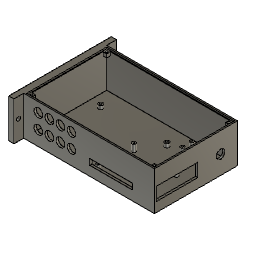
module_main v2 (Autodesk Fusion 360 design; units mm, degrees)
Autodesk Fusion 360 part; units mm, degrees
sketch "Sketch1" plane through (0, 0, 0) normal (0, 0, 1) x (1, 0, 0)
  line L0 (0, 0) -> (178, 0)
  line L1 (178, 0) -> (178, 113)
  line L2 (178, 113) -> (0, 113)
  line L3 (0, 113) -> (0, 0)
  dimension "d1" = 178
  dimension "d2" = 113
  constraint horizontal L0
  constraint vertical L1
  constraint horizontal L2
  constraint vertical L3
  constraint coincident L0.start L3.end
  measures "d1" distance of L0.start L0.end
  measures "d2" distance of L0.start L2.end
extrude "Extrude1" add sketch "Sketch1" along normal blind 3
extrude "Extrude2" add 1 faces at (59.3333, 37.6667, 3) along direction (0, 0, 1) blind 50 thin wall 3 inside
sketch "Sketch2" plane through (0, 0, 0) normal (-1, 0, 0) x (0, -1, 0)
  line L0 (-113, 0) -> (0, 0)
  line L1 (0, 0) -> (0, 53)
  line L2 (0, 53) -> (-113, 53)
  line L3 (-113, 53) -> (-113, 0)
  line L4 (13.35, 0) -> (-126.35, 0)
  line L5 (-126.35, 0) -> (-126.35, 53)
  line L6 (-126.35, 53) -> (13.35, 53)
  line L7 (13.35, 53) -> (13.35, 0)
  line L8 (13.35, 0) -> (-126.35, 53) construction
  line L9 (-126.35, 0) -> (13.35, 53) construction
  point P0 (-56.5, 26.5)
  dimension "d8" = 139.7
  dimension "d9" = 53
  constraint horizontal L4
  constraint perpendicular L4 L5
  constraint parallel L4 L6
  constraint parallel L5 L7
  constraint coincident L8 P0
  constraint coincident L9 P0
  measures "d8" distance of L5.end L6.end
  measures "d9" distance of L4.end L5.end
extrude "Extrude3" add sketch "Sketch2" along normal blind 7
sketch "Sketch3" plane through (-7, 0, 0) normal (-1, 0, 0) x (0, -1, 0)
  line L0 (13.35, 53) -> (-126.35, 53)
  line L1 (-126.35, 53) -> (-126.35, 0)
  line L2 (-126.35, 0) -> (13.35, 0)
  line L3 (13.35, 0) -> (13.35, 53)
  point P0 (-120, 26.5)
  point P1 (7, 26.5)
hole "Hole1" at (-7, 120, 26.5) at (-7, -7, 26.5) direction (1, 0, 0) diameter 5.5 depth 12 tip angle 118
sketch "Sketch4" plane through (0, 0, 3) normal (0, 0, 1) x (-1, 0, 0)
  line L0 (-175, -110) -> (-3, -110)
  line L1 (-3, -110) -> (-3, -3)
  line L2 (-3, -3) -> (-175, -3)
  line L3 (-175, -3) -> (-175, -110)
  circle A0 centre (-151.5, -7.5) radius 2.5
  circle A1 centre (-151.5, -56.5) radius 2.5
  circle A2 centre (-93.5, -56.5) radius 2.5
  circle A3 centre (-93.5, -7.5) radius 2.5
  dimension "d15" = 5
  dimension "d16" = 5
  dimension "d17" = 5
  dimension "d18" = 5
  measures "d15" diameter of A0
  measures "d16" diameter of A1
  measures "d17" diameter of A2
  measures "d18" diameter of A3
extrude "Extrude4" add sketch "Sketch4" along normal blind 10 contours A0 | A1 | A2 | A3
hole "Hole3" at (93.5, 56.5, 13) direction (0, 0, -1) diameter 2 depth 4 tip angle 118
hole "Hole4" at (151.5, 56.5, 13) direction (0, 0, -1) diameter 2 depth 4 tip angle 118
hole "Hole5" at (151.5, 7.5, 13) direction (0, 0, -1) diameter 2 depth 4 tip angle 118
hole "Hole6" at (93.5, 7.5, 13) direction (0, 0, -1) diameter 2 depth 4 tip angle 118
sketch "Sketch6" plane through (178, 0, 0) normal (1, 0, 0) x (0, 1, 0)
  line L0 (0, 0) -> (113, 0)
  line L1 (113, 0) -> (113, 53)
  line L2 (113, 53) -> (0, 53)
  line L3 (0, 53) -> (0, 0)
  line L4 (3, 13) -> (59, 13)
  line L5 (59, 13) -> (59, 31)
  line L6 (59, 31) -> (3, 31)
  line L7 (3, 31) -> (3, 13)
  point P0 (3, 13)
  dimension "d38" = 56
  dimension "d39" = 18
  constraint horizontal L4
  constraint vertical L5
  constraint horizontal L6
  constraint vertical L7
  constraint coincident P0 L4.start
  measures "d38" distance of P0 L4.end
  measures "d39" distance of P0 L6.end
extrude "Extrude5" cut sketch "Sketch6" against normal blind 4 contours L4 L5 L6 L7
sketch "Sketch7" plane through (0, 0, 0) normal (0, -1, 0) x (1, 0, 0)
  line L0 (0, 0) -> (178, 0)
  line L1 (178, 0) -> (178, 53)
  line L2 (178, 53) -> (0, 53)
  line L3 (0, 53) -> (0, 0)
  line L4 (148, 13) -> (90, 13)
  line L5 (90, 13) -> (90, 21)
  line L6 (90, 21) -> (148, 21)
  line L7 (148, 21) -> (148, 13)
  point P0 (148, 13)
  dimension "d42" = 58
  dimension "d43" = 8
  constraint horizontal L4
  constraint vertical L5
  constraint horizontal L6
  constraint vertical L7
  constraint coincident P0 L4.start
  measures "d42" distance of P0 L4.end
  measures "d43" distance of P0 L6.end
extrude "Extrude6" cut sketch "Sketch7" against normal blind 4 contours L4 L5 L6 L7
sketch "Sketch8" plane through (0, 0, 3) normal (0, 0, 1) x (-1, 0, 0)
  circle A0 centre (-151.5, -7.5) radius 2.5
  circle A1 centre (-151.5, -56.5) radius 2.5
  circle A2 centre (-93.5, -7.5) radius 2.5
  circle A3 centre (-93.5, -56.5) radius 2.5
  line L0 (-175, -110) -> (-3, -110)
  line L1 (-3, -110) -> (-3, -3)
  line L2 (-3, -3) -> (-175, -3)
  line L3 (-175, -3) -> (-175, -110)
  circle A4 centre (-131.18, -97.7) radius 2.5
  circle A5 centre (-151.5, -97.7) radius 2.5
  circle A6 centre (-151.5, -85) radius 2.5
  circle A7 centre (-131.18, -85) radius 2.5
  point P0 (-151.5, -97.7)
  point P1 (-151.5, -85)
  point P2 (-131.18, -85)
  point P3 (-131.18, -97.7)
  dimension "d46" = 5
  dimension "d47" = 5
  dimension "d48" = 5
  dimension "d49" = 5
  constraint vertical P0 P1
  constraint horizontal P1 P2
  constraint vertical P2 P3
  constraint coincident P3 A4.centre
  constraint coincident P0 A5.centre
  constraint coincident P1 A6.centre
  constraint coincident P2 A7.centre
  measures "d46" diameter of A4
  measures "d47" diameter of A5
  measures "d48" diameter of A6
  measures "d49" diameter of A7
extrude "Extrude7" add sketch "Sketch8" along normal blind 10 contours A4 | A5 | A6 | A7
hole "Hole7" at (131.18, 97.7, 13) direction (0, 0, -1) diameter 2 depth 4 tip angle 180
hole "Hole8" at (131.18, 85, 13) direction (0, 0, -1) diameter 2 depth 4 tip angle 180
hole "Hole9" at (151.5, 97.7, 13) direction (0, 0, -1) diameter 2 depth 4 tip angle 180
hole "Hole10" at (151.5, 85, 13) direction (0, 0, -1) diameter 2 depth 4 tip angle 180
sketch "Sketch9" plane through (178, 0, 0) normal (1, 0, 0) x (0, 1, 0)
  line L0 (59, 13) -> (3, 13)
  line L1 (3, 13) -> (3, 31)
  line L2 (3, 31) -> (59, 31)
  line L3 (59, 31) -> (59, 13)
  line L4 (0, 0) -> (113, 0)
  line L5 (113, 0) -> (113, 53)
  line L6 (113, 53) -> (0, 53)
  line L7 (0, 53) -> (0, 0)
  circle A0 centre (90, 25) radius 6
  dimension "d64" = 12
  measures "d64" diameter of A0
extrude "Extrude8" cut sketch "Sketch9" against normal blind 4 contours A0
sketch "Sketch10" plane through (0, 0, 3) normal (0, 0, 1) x (-1, 0, 0)
  circle A0 centre (-151.5, -85) radius 2.5
  circle A1 centre (-131.18, -97.7) radius 2.5
  circle A2 centre (-131.18, -85) radius 2.5
  circle A3 centre (-151.5, -97.7) radius 2.5
  circle A4 centre (-151.5, -7.5) radius 2.5
  circle A5 centre (-151.5, -56.5) radius 2.5
  circle A6 centre (-93.5, -7.5) radius 2.5
  circle A7 centre (-93.5, -56.5) radius 2.5
  line L0 (-175, -110) -> (-3, -110)
  line L1 (-3, -110) -> (-3, -3)
  line L2 (-3, -3) -> (-175, -3)
  line L3 (-175, -3) -> (-175, -110)
  circle A8 centre (-110, -85) radius 3
  circle A9 centre (-20, -85) radius 3
  dimension "d67" = 6
  dimension "d68" = 6
  measures "d67" diameter of A8
  measures "d68" diameter of A9
extrude "Extrude9" add sketch "Sketch10" along normal blind 5 contours A8 | A9
hole "Hole11" at (110, 85, 8) direction (0, 0, -1) diameter 2.75 depth 4 tip angle 180
hole "Hole12" at (20, 85, 8) direction (0, 0, -1) diameter 2.75 depth 4 tip angle 180
sketch "Sketch11" plane through (0, 0, 0) normal (0, -1, 0) x (1, 0, 0)
  line L0 (90, 13) -> (90, 21)
  line L1 (90, 21) -> (148, 21)
  line L2 (148, 21) -> (148, 13)
  line L3 (148, 13) -> (90, 13)
  line L4 (0, 0) -> (178, 0)
  line L5 (178, 0) -> (178, 53)
  line L6 (178, 53) -> (0, 53)
  line L7 (0, 53) -> (0, 0)
  circle A0 centre (20, 20) radius 6
  circle A1 centre (35, 20) radius 6
  circle A2 centre (50, 20) radius 6
  circle A3 centre (65, 20) radius 6
  circle A4 centre (20, 40) radius 6
  circle A5 centre (35, 40) radius 6
  circle A6 centre (50, 40) radius 6
  circle A7 centre (65, 40) radius 6
  dimension "d77" = 12
  dimension "d78" = 12
  dimension "d79" = 12
  dimension "d80" = 12
  dimension "d81" = 12
  dimension "d82" = 12
  dimension "d83" = 12
  dimension "d84" = 12
  measures "d77" diameter of A0
  measures "d78" diameter of A1
  measures "d79" diameter of A2
  measures "d80" diameter of A3
  measures "d81" diameter of A4
  measures "d82" diameter of A5
  measures "d83" diameter of A6
  measures "d84" diameter of A7
extrude "Extrude10" cut sketch "Sketch11" against normal blind 4 contours A0 | A1 | A2 | A3 | A4 | A5 | A6 | A7
sketch "Sketch12" plane through (0, 0, 53) normal (0, 0, 1) x (-1, 0, 0)
  line L0 (-3, -110) -> (-175, -110)
  line L1 (-175, -110) -> (-175, -3)
  line L2 (-175, -3) -> (-3, -3)
  line L3 (-3, -3) -> (-3, -110)
  line L4 (0, 0) -> (-178, 0)
  line L5 (-178, 0) -> (-178, -113)
  line L6 (-178, -113) -> (0, -113)
  line L7 (0, -113) -> (0, -126.35)
  line L8 (0, -126.35) -> (7, -126.35)
  line L9 (7, -126.35) -> (7, 13.35)
  line L10 (7, 13.35) -> (0, 13.35)
  line L11 (0, 13.35) -> (0, 0)
  line L12 (-2, -111) -> (-176, -111)
  line L13 (-176, -111) -> (-176, -2)
  line L14 (-176, -2) -> (-2, -2)
  line L15 (-2, -2) -> (-2, -111)
  constraint horizontal L12
  constraint vertical L13
  constraint horizontal L14
  constraint vertical L15
extrude "Extrude11" cut sketch "Sketch12" against normal blind 2 contours L12 L13 L14 L15
ref_plane "WorkPlane1" through (85.5, 56.5, 51) normal (0, 0, 1) x (1, 0, 0)
sketch "Sketch13" plane through (0, 0, 51) normal (0, 0, 1) x (1, 0, 0)
  line L0 (3, 3) -> (8, 3)
  line L1 (8, 3) -> (8, 8)
  line L2 (8, 8) -> (3, 8)
  line L3 (3, 8) -> (3, 3)
  line L4 (3, 110) -> (8, 110)
  line L5 (8, 110) -> (8, 105)
  line L6 (8, 105) -> (3, 105)
  line L7 (3, 105) -> (3, 110)
  line L8 (175, 3) -> (170, 3)
  line L9 (170, 3) -> (170, 8)
  line L10 (170, 8) -> (175, 8)
  line L11 (175, 8) -> (175, 3)
  line L12 (175, 110) -> (170, 110)
  line L13 (170, 110) -> (170, 105)
  line L14 (170, 105) -> (175, 105)
  line L15 (175, 105) -> (175, 110)
  dimension "d90" = 5
  dimension "d91" = 5
  dimension "d92" = 5
  dimension "d93" = 5
  dimension "d94" = 5
  dimension "d95" = 5
  dimension "d96" = 5
  dimension "d97" = 5
  constraint horizontal L0
  constraint vertical L1
  constraint horizontal L2
  constraint vertical L3
  constraint horizontal L4
  constraint vertical L5
  constraint horizontal L6
  constraint vertical L7
  constraint horizontal L8
  constraint vertical L9
  constraint horizontal L10
  constraint vertical L11
  constraint horizontal L12
  constraint vertical L13
  constraint horizontal L14
  constraint vertical L15
  measures "d90" distance of L0.start L0.end
  measures "d91" distance of L0.start L2.end
  measures "d92" distance of L4.start L4.end
  measures "d93" distance of L4.start L6.end
  measures "d94" distance of L8.start L8.end
  measures "d95" distance of L8.start L10.end
  measures "d96" distance of L12.start L12.end
  measures "d97" distance of L12.start L14.end
extrude "Extrude12" add sketch "Sketch13" against normal blind 5
sketch "Sketch14" plane through (0, 0, 51) normal (0, 0, 1) x (-1, 0, 0)
  line L0 (-8, -3) -> (-8, -8)
  line L1 (-8, -8) -> (-3, -8)
  line L2 (-3, -8) -> (-3, -105)
  line L3 (-3, -105) -> (-8, -105)
  line L4 (-8, -105) -> (-8, -110)
  line L5 (-8, -110) -> (-170, -110)
  line L6 (-170, -110) -> (-170, -105)
  line L7 (-170, -105) -> (-175, -105)
  line L8 (-175, -105) -> (-175, -8)
  line L9 (-175, -8) -> (-170, -8)
  line L10 (-170, -8) -> (-170, -3)
  line L11 (-170, -3) -> (-8, -3)
  line L12 (-2, -2) -> (-176, -2)
  line L13 (-176, -2) -> (-176, -111)
  line L14 (-176, -111) -> (-2, -111)
  line L15 (-2, -111) -> (-2, -2)
  point P0 (-5.5, -5.5)
  point P1 (-5.5, -107.5)
  point P2 (-172.5, -107.5)
  point P3 (-172.5, -5.5)
hole "Hole13" at (172.5, 5.5, 51) at (5.5, 107.5, 51) at (5.5, 5.5, 51) at (172.5, 107.5, 51) direction (0, 0, -1) diameter 2.75 depth 6 tip angle 180
